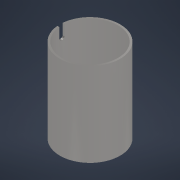
# Autodesk Inventor part: 025
Saved by Autodesk Inventor 2022 (Build 260153000, 153)
## iProperties
Created: 2021-11-04
Part Number: 025
Material: Steel, Carbon
Document SubType Name: Modeling
Designer: vinicius.miguel
Density: 7.85 g/cm^3
Appearance: Semi-Polished
Mass: 996.175 g
Surface Area: 901.746 cm^2
Volume: 126.901 cm^3
Author: vinicius.miguel
Autodesk Inventor part; units mm, degrees
ref_plane "XZ Plane" through (0, 0, 0) normal (0, 1, 0) x (-1, 0, 0)
ref_plane "XY Plane" through (0, 0, 0) normal (0, 0, 1) x (1, 0, 0)
sketch "Sketch1" plane through (0, 0, 0) normal (0, 1, 0) x (-1, 0, 0)
  circle A0 centre (0, 0) radius 44.45
  circle A1 centre (0, 0) radius 41.55
  dimension "d0" = 88.9
  dimension "d1" = 2.9
  constraints: 2 centre point, 1 coincident
  measures "d0" diameter of A0
  measures "d1" radial gap between concentric circles of A0 A1
extrude "Extrusion1" add sketch "Sketch1" along normal blind 124
ref_plane "Work Plane1" through (-44.45, 0, 0) normal (1, 0, 0) x (0, 1, 0)
sketch "Sketch2" plane through (-44.45, 0, 0) normal (1, 0, 0) x (0, 1, 0)
  circle A0 centre (15, 0) radius 4
  line L0 (0, -44.45) -> (0, 44.45) projected
  line L1 (15, -4) -> (0, -4)
  line L2 (15, 4) -> (0, 4)
  line L3 (124, -44.45) -> (124, 44.45) projected
  circle A1 centre (109, 0) radius 4
  line L4 (109, -4) -> (124, -4)
  line L5 (109, 4) -> (124, 4)
  point P0 (0, 0)
  dimension "d16" = 8
  dimension "d17" = 15
  dimension "d18" = 15
  constraints: 8 end point, 4 point on circle, 4 point on line, 3 horizontal alignment, 3 perpendicular, 2 centre point, 2 tangent, 1 equal radius, 1 horizontal
  measures "d16" diameter of A0
  measures "d17" distance of A0.centre point (0, 0)
  measures "d18" distance from line of L3 A1.centre
extrude "Extrusion2" cut sketch "Sketch2" along normal blind 50
equation "\"d18\" = d17"
body "Solid1"
